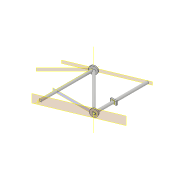
# Autodesk Inventor part: 00_Beam_Ocular_Detectoin
Saved by Autodesk Inventor 2019 (Build 230136000, 136)
## iProperties
Created: 2019-11-14
Part Number: 00_Beam_Ocular_Detectoin
Material: Generic
Document SubType Name: Modeling
Designer: diederichbenedict
Density: 1 g/cm^3
Appearance: Default
Author: diederichbenedict
Autodesk Inventor part; units mm, degrees
ref_plane "XZ Plane" through (0, 0, 0) normal (0, 1, 0) x (-1, 0, 0)
ref_plane "XY Plane" through (0, 0, 0) normal (0, 0, 1) x (1, 0, 0)
sketch "Sketch1" plane through (0, 0, 0) normal (0, 0, 1) x (1, 0, 0)
  circle A0 centre (0, 0) radius 1
  dimension "d0" = 2
  constraints: 1 centre point, 1 coincident
  measures "d0" diameter of A0
extrude "Extrusion1" add sketch "Sketch1" against normal blind 40
ref_plane "Work Plane1" through (0, 0, -40) normal (0, 0, -1) x (-1, 0, 0)
ref_plane "Work Plane3" through (0, 0, -40) normal (0.7071, 0, 0.7071) x (0, -1, 0)
ref_plane "Work Plane2" through (0, 0, -40) normal (1, 0, 0) x (0, 1, 0)
sketch "Sketch2" plane through (0, 0, -40) normal (0.7071, 0, 0.7071) x (0, -1, 0)
  ellipse E0 centre (0, 0) end of major axis (-1, 0) minor radius 0.7071 projected
  circle A0 centre (0, 0) radius 1
  point P0 (0, -28.2843)
  constraints: 1 centre point, 1 coincident, 1 other
extrude "Extrusion2" add sketch "Sketch2" along normal blind 40
ref_plane "Work Plane4" through (28.2843, 0, -11.7157) normal (0, 0, -1) x (-1, 0, 0)
sketch "Sketch3" plane through (28.2843, 0, -11.7157) normal (0, 0, -1) x (-1, 0, 0)
  ellipse E0 centre (0, 0) end of major axis (0, 1) minor radius 0.7071 projected
  circle A0 centre (0, 0) radius 1
  point P0 (28.2843, 0)
  constraints: 1 centre point, 1 coincident, 2 other
extrude "Extrusion3" add sketch "Sketch3" along normal blind 40
ref_plane "Work Plane5" through (0, 0, -40) normal (0.3827, 0, 0.9239) x (0, -1, 0)
sketch "Sketch4" plane through (0, 0, -40) normal (0.3827, 0, 0.9239) x (0, -1, 0)
  circle A0 centre (0, 0) radius 2.8545
  point P0 (0, -15.3073)
  constraints: 1 centre point
extrude "Extrusion4" add sketch "Sketch4" along normal blind 1
ref_plane "Work Plane6" through (28.2843, 0, -11.7157) normal (0.3827, 0, 0.9239) x (0.9239, 0, -0.3827)
sketch "Sketch5" plane through (28.2843, 0, -11.7157) normal (0.3827, 0, 0.9239) x (0.9239, 0, -0.3827)
  circle A0 centre (0, 0) radius 2.6859
  point P0 (-30.6147, 0)
  constraints: 1 centre point, 1 coincident
extrude "Extrusion5" add sketch "Sketch5" against normal blind 1
ref_plane "Work Plane7" through (28.2843, 0, -26.2157) normal (0, 0, -1) x (-1, 0, 0)
sketch "Sketch6" plane through (28.2843, 0, -26.2157) normal (0, 0, -1) x (-1, 0, 0)
  ellipse E0 centre (0, 0) end of major axis (0, 2.6859) minor radius 2.4814 projected
  line L0 (-2.1727, -1.2973) -> (2.1727, -1.2973)
  line L1 (2.1727, -1.2973) -> (2.1727, 1.2973)
  line L2 (2.1727, 1.2973) -> (-2.1727, 1.2973)
  line L3 (-2.1727, 1.2973) -> (-2.1727, -1.2973)
  line L4 (0, -1) -> (0, 1) projected
  line L5 (-2.1727, -1.2973) -> (2.1727, 1.2973) construction
  line L6 (2.1727, -1.2973) -> (-2.1727, 1.2973) construction
  point P0 (28.2843, 0)
  point P1 (0, 0)
  constraints: 12 end point, 3 midpoint, 2 parallel, 1 horizontal, 1 perpendicular, 2 other
extrude "Extrusion6" add sketch "Sketch6" along normal blind 1 contours L2 L1 L0 L3
body "Solid1"
